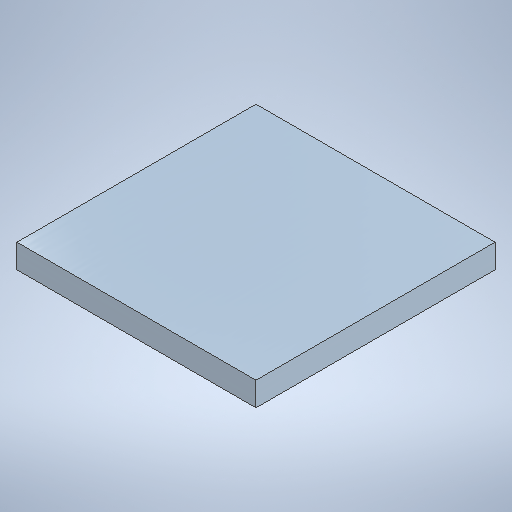
# Autodesk Inventor part: Mesa
Saved by Autodesk Inventor 2026 (Build 300175050, 175E)
## iProperties
Created: 2025-06-30
Part Number: Mesa
Material: Genérico
Document SubType Name: Modeling
Designer: piero
Density: 1 g/cm^3
Appearance: Valor por defecto
Author: piero
Autodesk Inventor part; units mm, degrees
ref_plane "YZ Plane" through (0, 0, 0) normal (1, 0, 0) x (0, 1, 0)
ref_plane "XZ Plane" through (0, 0, 0) normal (0, 1, 0) x (-1, 0, 0)
ref_plane "XY Plane" through (0, 0, 0) normal (0, 0, 1) x (1, 0, 0)
sketch "Boceto1" plane through (0, 0, 0) normal (0, 1, 0) x (-1, 0, 0)
  line L0 (0, 0) -> (400, 0)
  line L1 (400, 0) -> (400, -400)
  line L2 (400, -400) -> (0, -400)
  line L3 (0, -400) -> (0, 0)
  dimension "d0" = 400
  dimension "d1" = 400
  constraints: 8 end point, 2 parallel, 1 horizontal, 1 perpendicular
  measures "d0" distance of L1.end L2.end
  measures "d1" distance of L0.end L1.end
extrude "Extrusión1" add sketch "Boceto1" along normal blind 40
